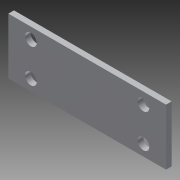
# Autodesk Inventor part: M - Upper Rail Connector Plate 1
Saved by Autodesk Inventor 2013 (Build 170138000, 138)
## iProperties
Created: 2013-02-17
Part Number: M - Upper Rail Connector Plate 1
Material: Aluminum 6061
Document SubType Name: Modeling
Designer: Moses
Density: 2.71 g/cm^3
Mass: 23.1072 g
Surface Area: 64.0074 cm^2
Volume: 8.52666 cm^3
Author: Moses
Autodesk Inventor part; units mm, degrees
ref_plane "YZ Plane" through (0, 0, 0) normal (1, 0, 0) x (0, 1, 0)
ref_plane "XZ Plane" through (0, 0, 0) normal (0, 1, 0) x (-1, 0, 0)
ref_plane "XY Plane" through (0, 0, 0) normal (0, 0, 1) x (1, 0, 0)
sketch "Sketch1" plane through (0, 0, 0) normal (0, 0, 1) x (1, 0, 0)
  line L0 (0, 0) -> (88.9, 0)
  line L1 (88.9, 0) -> (88.9, 31.75)
  line L2 (88.9, 31.75) -> (0, 31.75)
  line L3 (0, 31.75) -> (0, 0)
  circle A0 centre (12.7, 25.4) radius 3.302
  circle A1 centre (76.2, 25.4) radius 3.302
  circle A2 centre (12.7, 6.35) radius 3.302
  circle A3 centre (76.2, 6.35) radius 3.302
  line L4 (12.7, 25.4) -> (76.2, 25.4) construction
  line L5 (44.45, 31.75) -> (44.45, 0) construction
  point P0 (44.45, 25.4)
  dimension "d0" = 88.9
  dimension "d2" = 31.75
  dimension "d5" = 63.5
  dimension "d8" = 19.05
  dimension "d11" = 6.35
  dimension "d12" = 6.604
  constraints: 12 end point, 4 centre point, 3 midpoint, 2 horizontal, 2 parallel, 2 perpendicular, 1 point on line, 1 vertical, 6 other
  measures "d0" distance of L1.end L2.end
  measures "d2" distance of L2.end L0.start
  measures "d5" distance of L4.start L4.end
  measures "d8" distance of L4.start A2.centre
  measures "d11" distance from line of L2 L4.start
  measures "d12" diameter of A0
extrude "Extrusion1" add sketch "Sketch1" along normal blind 3.175
body "Solid1"
